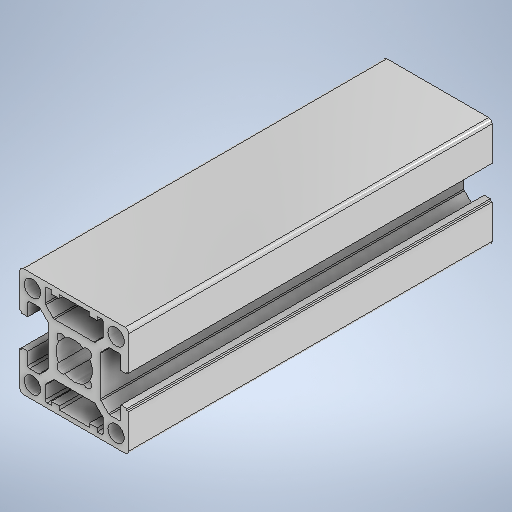
# Autodesk Inventor part: Perfil 30×30 2 rasgos opostos_001
Saved by Autodesk Inventor 2026 (Build 300175000, 175)
## iProperties
Created: 2025-04-05
Part Number: Perfil 30×30 2 rasgos opostos_001
Material: Aluminum 6061
Document SubType Name: Modeling
Designer: Tony Dias
Density: 2.7 g/cm^3
Appearance: Aluminum - Polished
Author: Tony Dias
Autodesk Inventor part; units mm, degrees
sketch "Sketch1" plane through (0, 0, 0) normal (0, 0, 1) x (1, 0, 0)
  circle A0 centre (0, 0) radius 5 construction
  line L0 (-15, 15) -> (0, 0) construction
  circle A1 centre (-3.5355, 3.5355) radius 1.25 construction
  circle A2 centre (-3.5355, -3.5355) radius 1.25 construction
  circle A3 centre (3.5355, -3.5355) radius 1.25 construction
  circle A4 centre (3.5355, 3.5355) radius 1.25 construction
  circle A5 centre (-11.5, 11.5) radius 2.25
  line L1 (-15, 15) -> (-15, 4.1) construction
  line L2 (-12.8, 4.1) -> (-15, 4.1) construction
  line L3 (-12.8, 8) -> (-9.5556, 8)
  line L4 (-12.8, 8) -> (-12.8, 4.1)
  line L5 (-7.2, 7.2) -> (0, 7.2) construction
  line L6 (-7.2, 7.2) -> (-7.2, 0) construction
  line L7 (-9.5556, 8) -> (-7.2, 5.6444)
  line L8 (-15, 15) -> (0, 15)
  line L9 (-8, 9.5556) -> (-5.6444, 7.2)
  line L10 (-5.6444, 7.2) -> (0, 7.2)
  arc A6 (-2.5481, 4.302) -> (-4.302, 2.5481) centre (-3.5355, 3.5355) ccw
  line L11 (0, 7.2) -> (0, 5)
  line L12 (-7.2, 5.6444) -> (-7.2, 0)
  line L13 (-8, 15) -> (-8, 8) construction
  line L14 (-8, 13.75) -> (-8, 9.5556)
  line L15 (-6.3, 12.8) -> (-4.1, 12.8)
  line L16 (-6.3, 13.75) -> (-6.3, 12.8)
  line L17 (-4.1, 13.75) -> (-4.1, 12.8)
  line L18 (-8, 13.75) -> (-6.3, 13.75)
  line L19 (-4.1, 13.75) -> (0, 13.75)
  line L20 (0, 15) -> (0, 13.75)
  line L21 (-15, 4.1) -> (-14.5, 4.1) construction
  line L22 (-14.5, 4.1) -> (-14.5, 4.6)
  line L23 (-14.5, 4.6) -> (-15, 4.6)
  line L24 (-15, 4.6) -> (-15, 4.1) construction
  line L25 (-14.5, 4.1) -> (-12.8, 4.1)
  line L26 (-7.2, 0) -> (-5, 0)
  line L27 (-15, 15) -> (-15, 4.6)
  arc A7 (0, 5) -> (-2.5481, 4.302) centre (0, 0) ccw
  arc A8 (-4.302, 2.5481) -> (-5, 0) centre (0, 0) ccw
  point P0 (-7.5, 7.5)
  dimension "d0" = 10
  dimension "d3" = 15
  dimension "d4" = 2.5
  dimension "d7" = 360
  dimension "d9" = 4.5
  dimension "d10" = 11.5
  dimension "d11" = 11.5
  dimension "d12" = 15
  dimension "d13" = 4.1
  dimension "d14" = 2.2
  dimension "d15" = 1.25
  dimension "d16" = 2.2
  dimension "d18" = 1.1
  dimension "d19" = 1.25
  dimension "d20" = 2.2
  dimension "d22" = 2.2
  dimension "d23" = 0.5
  dimension "d24" = 4.1
  constraints: 56 end point, 13 point on circle, 10 horizontal, 9 centre point, 8 vertical, 7 point on line, 4 coincident, 4 vertical alignment, 3 collinear, 3 concentric, 3 horizontal alignment, 3 parallel, 3 perpendicular, 1 midpoint, 10 other
  measures "d0" diameter of A0
  measures "d3" horizontal distance of point (0, 0) L0.start
  measures "d4" diameter of A1
  measures "d9" diameter of A5
  measures "d10" horizontal distance of point (0, 0) A5.centre
  measures "d11" horizontal distance of point (0, 0) A5.centre
  measures "d12" horizontal distance of L0.start point (0, 0)
  measures "d13" vertical distance of point (0, 0) L1.end
  measures "d14" distance of L2.start L1.end
  measures "d15" distance edge to line of A5 L3
  measures "d16" distance edge to line of A0 L5
  measures "d18" distance from line of point (-7.5, 7.5) L7
  measures "d19" distance from line of L8 L14.start
  measures "d20" distance of L15.start L15.end
  measures "d22" distance between parallel lines of L8 L15
  measures "d23" distance of L22.end L23.end
  measures "d24" horizontal distance of point (0, 0) L15.end
extrude "Extrusion1" add sketch "Sketch1" along normal mid plane 100
mirror "Mirror1" about plane through (0, 0, 0) normal (1, 0, 0) of "Extrusion1"
mirror "Mirror2" about plane through (0, 0, 0) normal (0, 1, 0) of "Extrusion1", "Mirror1"
fillet "Fillet1" radius 1 4 edges at (-15, 15, 0) (15, 15, 0) (15, -15, 0) (-15, -15, 0)
fillet "Fillet2" radius 0.5 23 edges at (-7.2, -5.6444, 0) (-9.5556, -8, 0) (-5.6444, 7.2, 0) (5.6444, 7.2, 0) (8, 9.5556, 0) (-12.8, -8, 0) (-7.2, 5.6444, 0) (-9.5556, 8, 0) (-12.8, 8, 0) (-5.6444, -7.2, 0) (-8, -9.5556, 0) (5.6444, -7.2, 0) (8, -9.5556, 0) (-8, -13.75, 0) (8, -13.75, 0) (9.5556, -8, 0) (7.2, -5.6444, 0) (12.8, -8, 0) (-8, 13.75, 0) (8, 13.75, 0) (7.2, 5.6444, 0) (9.5556, 8, 0) (12.8, 8, 0)
fillet "Fillet3" radius 0.5 1 edges at (-8, 9.5556, 0)
equation "\"d19\" = d15"
equation "\"d20\" = d14"
equation "\"d22\" = d14"
body "Solid1"
